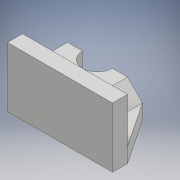
# Autodesk Inventor part: 28
Saved by Autodesk Inventor 2017 (Build 210142000, 142)
## iProperties
Part Number: 28
Material: 一般
Document SubType Name: Modeling
Designer: Brian
Density: 1 g/cm^3
Appearance: 預設
Author: Brian
Autodesk Inventor part; units mm, degrees
ref_plane "YZ Plane" through (0, 0, 0) normal (1, 0, 0) x (0, 1, 0)
ref_plane "XZ Plane" through (0, 0, 0) normal (0, 1, 0) x (-1, 0, 0)
ref_plane "XY Plane" through (0, 0, 0) normal (0, 0, 1) x (1, 0, 0)
sketch "草圖1" plane through (0, 0, 0) normal (0, 1, 0) x (-1, 0, 0)
  line L0 (0, 0) -> (-70, 0)
  line L1 (-70, 0) -> (-70, -40)
  line L2 (-70, -40) -> (0, -40)
  line L3 (0, -40) -> (0, 0)
  dimension "d0" = 40
  dimension "d1" = 70
  constraints: 8 end point, 2 parallel, 1 horizontal, 1 perpendicular
  measures "d0" distance of L2.end L0.start
  measures "d1" distance of L1.end L2.end
extrude "擠出1" add sketch "草圖1" along normal blind 10
sketch "草圖2" plane through (0, 10, 0) normal (0, 1, 0) x (1, 0, 0)
  line L0 (0, 40) -> (0, 0) projected
  line L1 (0, 40) -> (40, 40)
  line L2 (40, 40) -> (40, 20)
  line L3 (40, 20) -> (0, 20)
  line L4 (0, 20) -> (0, 40)
  line L5 (40, 40) -> (70, 40)
  line L6 (70, 40) -> (70, 30)
  line L7 (70, 30) -> (40, 30)
  line L8 (40, 30) -> (40, 40)
  dimension "d4" = 30
  dimension "d5" = 40
  dimension "d6" = 20
  dimension "d7" = 10
  constraints: 16 end point, 4 parallel, 2 horizontal, 2 perpendicular
  measures "d4" distance of L6.end L7.end
  measures "d5" distance of L2.end L3.end
  measures "d6" distance between parallel lines of L1 L3
  measures "d7" distance between parallel lines of L5 L7
extrude "擠出2" add sketch "草圖2" along normal blind 30
chamfer "倒角1" distance 10 angle 45 1 edges at (40, 25, -30)
chamfer "倒角2" distance 20 distance2 30 1 edges at (70, 40, -35) measured on face at (13.3333, 40, -26.6668)
sketch "草圖3" plane through (0, 10, -20) normal (0, 0, 1) x (1, 0, 0)
  line L0 (0, 30) -> (40, 30) projected
  circle A0 centre (20, 30) radius 10
  point P0 (0, -10)
  dimension "d16" = 20
  constraints: 1 centre point, 1 midpoint
  measures "d16" diameter of A0
extrude "擠出3" cut sketch "草圖3" against normal blind 30
